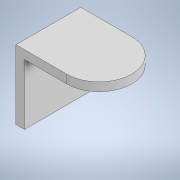
# Autodesk Inventor part: turret y top
Saved by Autodesk Inventor 2020 (Build 240168000, 168)
## iProperties
Created: 2019-06-21
Part Number: turret y top
Material: Generic
Document SubType Name: Modeling
Designer: kangh
Density: 1 g/cm^3
Appearance: Default
Author: kangh
Autodesk Inventor part; units mm, degrees
ref_plane "YZ Plane" through (0, 0, 0) normal (1, 0, 0) x (0, 1, 0)
ref_plane "XZ Plane" through (0, 0, 0) normal (0, 1, 0) x (-1, 0, 0)
ref_plane "XY Plane" through (0, 0, 0) normal (0, 0, 1) x (1, 0, 0)
sketch "Sketch1" plane through (0, 0, 0) normal (0, 1, 0) x (-1, 0, 0)
  circle A0 centre (0, 0) radius 19.05
  circle A1 centre (0, 0) radius 12.7
  circle A2 centre (0, 0) radius 4
  line L0 (12.7, 0) -> (11.2, 0)
  circle A3 centre (11.2, 0) radius 1.5
  line L1 (11.2, 1.5) -> (2.3814, 3.2139)
  line L2 (11.2, -1.5) -> (2.3814, -3.2139)
  circle A4 centre (0, 11.2) radius 1.5
  line L3 (-1.5, 11.2) -> (-3.2139, 2.3814)
  line L4 (1.5, 11.2) -> (3.2139, 2.3814)
  circle A5 centre (-11.2, 0) radius 1.5
  line L5 (-11.2, -1.5) -> (-2.3814, -3.2139)
  line L6 (-11.2, 1.5) -> (-2.3814, 3.2139)
  circle A6 centre (0, -11.2) radius 1.5
  line L7 (1.5, -11.2) -> (3.2139, -2.3814)
  line L8 (-1.5, -11.2) -> (-3.2139, -2.3814)
  line L9 (0, -19.05) -> (29.9563, -19.05)
  line L10 (29.9563, -19.05) -> (29.9563, 19.05)
  line L11 (29.9563, 19.05) -> (0, 19.05)
  line L12 (0, 19.05) -> (0, -19.05)
  point P0 (0, 12.7)
  point P1 (-12.7, 0)
  point P2 (0, -12.7)
  point P3 (-3.0784, -3.0784)
  point P4 (-3.0784, 3.0784)
  point P5 (3.0784, 3.0784)
  point P6 (3.0784, -3.0784)
  point P7 (0, 19.05)
  dimension "d2" = 38.1
  dimension "d3" = 25.4
  dimension "d4" = 8
  dimension "d5" = 1.5
  dimension "d6" = 360
  constraints: 26 end point, 14 point on circle, 5 centre point, 4 coincident, 2 horizontal, 2 parallel, 1 horizontal alignment, 1 perpendicular, 42 other
  measures "d4" diameter of A2
  measures "d5" distance of L0.start L0.end
extrude "Extrusion1" add sketch "Sketch1" along normal blind 2 contours A0 L12 A1 | A0 L11 L10 L9 | L12 A1 A0 | A4 L3 L6 A5 A1 | A1 A3 L1 L4 A4 | A6 L7 L2 A3 A1 | A1 A5 L5 L8 A6
sketch "Sketch2" plane through (0, 2, 0) normal (0, 1, 0) x (1, 0, 0)
  line L0 (0, 19.05) -> (-29.9563, 19.05) projected
  line L1 (-29.9563, -19.05) -> (0, -19.05)
  line L2 (0, -19.05) -> (0, 19.05)
  line L3 (0, 19.05) -> (-29.9563, 19.05)
  line L4 (-29.9563, 19.05) -> (-29.9563, -19.05)
  circle A0 centre (0, 0) radius 19.05
  point P0 (0, -19.05)
  constraints: 8 end point, 2 parallel, 1 centre point, 1 coincident, 1 horizontal, 1 perpendicular
extrude "Extrusion2" add sketch "Sketch2" along normal blind 3
sketch "Sketch3" plane through (0, 0, 0) normal (0, -1, 0) x (1, 0, 0)
  point P0 (0, 0)
sketch "Sketch4" plane through (0, 5, 0) normal (0, 1, 0) x (1, 0, 0)
  line L0 (-29.9563, -19.05) -> (-24.9563, -19.05)
  line L1 (-24.9563, -19.05) -> (-24.9563, 18.9252)
  line L2 (-24.9563, 18.9252) -> (-29.9563, 18.9252)
  line L3 (-29.9563, 18.9252) -> (-29.9563, -19.05)
  point P0 (0, 0)
  dimension "d11" = 5
  constraints: 8 end point, 2 parallel, 1 horizontal, 1 perpendicular
  measures "d11" distance of L2.end L1.end
extrude "Extrusion3" add sketch "Sketch4" against normal blind 40.64
body "Solid1"
